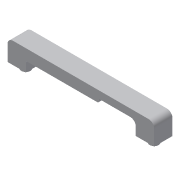
# Autodesk Inventor part: USB-Halter
Saved by Autodesk Inventor 2013 (Build 170138000, 138)
## iProperties
Created: 2013-08-23
Part Number: USB-Halter
Material: Allgemein
Document SubType Name: Modeling
Designer: Harald
Density: 1 g/cm^3
Author: Harald
Autodesk Inventor part; units mm, degrees
ref_plane "YZ Plane" through (0, 0, 0) normal (1, 0, 0) x (0, 1, 0)
ref_plane "XZ Plane" through (0, 0, 0) normal (0, 1, 0) x (-1, 0, 0)
ref_plane "XY Plane" through (0, 0, 0) normal (0, 0, 1) x (1, 0, 0)
sketch "Skizze1" plane through (0, 0, 0) normal (0, 0, 1) x (1, 0, 0)
  line L0 (0, 0) -> (10, 0)
  line L1 (10, 0) -> (10, 10)
  line L2 (10, 10) -> (0, 10)
  line L3 (0, 10) -> (0, 0)
  line L4 (70, 10) -> (80, 10)
  line L5 (80, 10) -> (80, 0)
  line L6 (80, 0) -> (70, 0)
  line L7 (70, 0) -> (70, 10)
  dimension "d0" = 10
  dimension "d1" = 10
  dimension "d2" = 10
  dimension "d3" = 10
  dimension "d4" = 60
  constraints: 16 end point, 4 parallel, 2 horizontal, 2 perpendicular, 1 collinear
  measures "d0" distance of L2.end L1.end
  measures "d1" distance of L1.end L0.end
  measures "d2" distance of L5.end L6.end
  measures "d3" distance of L4.end L5.end
  measures "d4" distance between parallel lines of L7 L1
extrude "Extrusion1" add sketch "Skizze1" along normal blind 7.5
sketch "Skizze2" plane through (0, 0, 7.5) normal (0, 0, 1) x (1, 0, 0)
  line L0 (80, 10) -> (70, 10) projected
  line L1 (70, 10) -> (70, 0) projected
  line L2 (70, 0) -> (80, 0) projected
  line L3 (80, 0) -> (80, 10) projected
  line L4 (0, 10) -> (80, 10)
  line L5 (80, 10) -> (80, 0)
  line L6 (80, 0) -> (0, 0)
  line L7 (0, 0) -> (0, 10)
  constraints: 8 end point, 2 parallel, 1 horizontal, 1 perpendicular
extrude "Extrusion2" add sketch "Skizze2" along normal blind 4
fillet "Rundung1" radius 3 1 edges at (0, 5, 11.5)
fillet "Rundung1" radius 3 1 edges at (80, 5, 11.5)
fillet "Rundung1" radius 3 1 edges at (70, 5, 7.5)
fillet "Rundung1" radius 3 1 edges at (10, 5, 7.5)
sketch "Skizze3" plane through (0, 0, 7.5) normal (0, 0, -1) x (-1, 0, 0)
  line L0 (0, 0) -> (-50, 0)
  line L1 (-50, 0) -> (-50, 2)
  line L2 (-50, 2) -> (0, 2)
  line L3 (0, 2) -> (0, 0)
  dimension "d13" = 50
  dimension "d14" = 2
  constraints: 8 end point, 2 parallel, 1 horizontal, 1 perpendicular
  measures "d13" distance of L1.end L2.end
  measures "d14" distance of L0.end L1.end
extrude "Extrusion3" add sketch "Skizze3" along normal blind 2
fillet "Rundung2" radius 1 1 edges at (50, 1, 5.5)
sketch "Skizze4" plane through (0, 0, 0) normal (0, 0, -1) x (-1, 0, 0)
  line L0 (0, 0) -> (-10, 0) projected
  line L1 (0, 10) -> (0, 0) projected
  circle A0 centre (-5, 5) radius 2.5
  dimension "d18" = 5
  dimension "d19" = 5
  dimension "d20" = 5
  constraints: 1 centre point
  measures "d18" diameter of A0
  measures "d19" distance from line of L1 A0.centre
  measures "d20" distance from line of L0 A0.centre
sketch "Skizze5" plane through (0, 0, 0) normal (0, 0, -1) x (-1, 0, 0)
  line L0 (-80, 0) -> (-70, 0) projected
  line L1 (-70, 0) -> (-70, 10) projected
  circle A0 centre (-75, 5) radius 2.5
  point P0 (0, 0)
  dimension "d21" = 5
  dimension "d22" = 5
  dimension "d23" = 5
  constraints: 1 centre point
  measures "d21" diameter of A0
  measures "d22" distance from line of L1 A0.centre
  measures "d23" distance from line of L0 A0.centre
extrude "Extrusion4" add sketch "Skizze4" along normal blind 3
extrude "Extrusion5" add sketch "Skizze5" along normal blind 3
